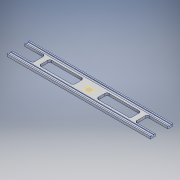
# Autodesk Inventor part: top
Saved by Autodesk Inventor 2017 (Build 210142000, 142)
## iProperties
Created: 2016-09-24
Part Number: top
Material: Aluminum 6061
Document SubType Name: Modeling
Designer: Kevin G
Density: 2.7 g/cm^3
Appearance: Aluminum - Flat
Author: Kevin G
Autodesk Inventor part; units mm, degrees
note: some values were not read from the file. Chosen so that the rebuilt part matches the saved one: direction of "Emboss7".
ref_plane "YZ Plane" through (0, 0, 0) normal (1, 0, 0) x (0, 1, 0)
ref_plane "XZ Plane" through (0, 0, 0) normal (0, 1, 0) x (-1, 0, 0)
ref_plane "XY Plane" through (0, 0, 0) normal (0, 0, 1) x (1, 0, 0)
sketch "Sketch1" plane through (0, 0, 0) normal (0, 0, 1) x (1, 0, 0)
  line L0 (-56.2006, 27.4418) -> (-175.6588, 27.4418)
  line L1 (-56.2006, -15.6625) -> (-175.6588, -15.6625)
  line L2 (-48.2006, -7.6625) -> (-48.2006, 19.4418)
  line L3 (-183.6588, -7.6625) -> (-183.6588, 19.4418)
  line L4 (-286.5288, -19.4915) -> (-213.2441, -19.4915)
  line L5 (-286.5288, 31.2885) -> (-213.2441, 31.2885)
  line L6 (-205.2441, 23.2885) -> (-205.2441, -11.4915)
  line L7 (51.9852, 27.4415) -> (171.5472, 27.4415)
  line L8 (51.9852, -15.6445) -> (171.5472, -15.6445)
  line L9 (43.9852, 19.4415) -> (43.9852, -7.6445)
  line L10 (179.5472, 19.4415) -> (179.5472, -7.6445)
  arc A0 (-205.2441, 23.2885) -> (-213.2441, 31.2885) centre (-213.2441, 23.2885) ccw
  arc A1 (-175.6588, 27.4418) -> (-183.6588, 19.4418) centre (-175.6588, 19.4418) ccw
  arc A2 (-183.6588, -7.6625) -> (-175.6588, -15.6625) centre (-175.6588, -7.6625) ccw
  arc A3 (-56.2006, -15.6625) -> (-48.2006, -7.6625) centre (-56.2006, -7.6625) ccw
  arc A4 (-48.2006, 19.4418) -> (-56.2006, 27.4418) centre (-56.2006, 19.4418) ccw
  arc A5 (-213.2441, -19.4915) -> (-205.2441, -11.4915) centre (-213.2441, -11.4915) ccw
  arc A6 (51.9852, 27.4415) -> (43.9852, 19.4415) centre (51.9852, 19.4415) ccw
  arc A7 (43.9852, -7.6445) -> (51.9852, -15.6445) centre (51.9852, -7.6445) ccw
  arc A8 (171.5472, -15.6445) -> (179.5472, -7.6445) centre (171.5472, -7.6445) ccw
  arc A9 (179.5472, 19.4415) -> (171.5472, 27.4415) centre (171.5472, 19.4415) ccw
  line L11 (-286.5288, 50.3385) -> (282.4312, 50.3385)
  line L12 (-286.5288, -38.5415) -> (282.4312, -38.5415)
  line L13 (-286.5288, 31.2885) -> (-286.5288, 50.3385)
  line L14 (-286.5288, -19.4915) -> (-286.5288, -38.5415)
  line L15 (179.5472, 5.8985) -> (201.1322, 5.9085)
  line L16 (282.4312, 31.2885) -> (209.1322, 31.2885)
  line L17 (201.1322, 23.2885) -> (201.1322, -11.4915)
  line L18 (209.1322, -19.4915) -> (282.4312, -19.4915)
  arc A10 (201.1322, -11.4915) -> (209.1322, -19.4915) centre (209.1322, -11.4915) ccw
  arc A11 (209.1322, 31.2885) -> (201.1322, 23.2885) centre (209.1322, 23.2885) ccw
  line L19 (282.4312, 50.3385) -> (282.4312, 31.2885)
  line L20 (282.4312, -19.4915) -> (282.4312, -38.5415)
  point P0 (0, 0)
  point P1 (0, 0)
  point P2 (-209.4751, 31.2885)
  point P3 (-205.2441, 26.6389)
  point P4 (-209.4751, -19.4915)
  point P5 (-179.9924, 27.4418)
  point P6 (-183.6588, 23.2495)
  point P7 (-183.6588, -11.4325)
  point P8 (-179.4288, -15.6625)
  point P9 (-48.2006, 23.2495)
  point P10 (-52.4306, 27.4418)
  point P11 (-52.9924, -15.6625)
  point P12 (-48.2006, -11.4325)
  point P13 (-205.2441, -15.2625)
  point P14 (48.2152, 27.4415)
  point P15 (43.9852, 23.2115)
  point P16 (48.2152, -15.6445)
  point P17 (179.5472, 23.2115)
  point P18 (175.3172, 27.4415)
  point P19 (175.3172, -15.6445)
  point P20 (179.5472, -11.4145)
  point P21 (43.9852, -11.4145)
  dimension "d0" = 135.4582
  dimension "d1" = 43.1043
  dimension "d4" = 21.5853
  dimension "d5" = 92.1858
  dimension "d8" = 8
  dimension "d9" = 8
  dimension "d10" = 8
  dimension "d50" = 50.7799
  dimension "d62" = 88.8799
  dimension "d63" = 19.05
  dimension "d64" = 50.7799
  constraints: 42 end point, 24 point on circle, 24 tangent, 20 point on line, 12 centre point, 9 vertical, 8 equal radius, 8 horizontal, 1 collinear, 1 midpoint, 1 perpendicular
  measures "d0" distance between parallel lines of L2 L3
  measures "d1" distance between parallel lines of L1 L0
  measures "d4" distance between parallel lines of L3 L6
  measures "d5" distance between parallel lines of L9 L2
  measures "d8" radius of A0
  measures "d9" radius of A1
  measures "d10" radius of A6
  measures "d50" distance between parallel lines of L5 L4
  measures "d62" distance between parallel lines of L12 L11
  measures "d63" distance between parallel lines of L11 L5
  measures "d64" distance between parallel lines of L16 L18
ref_plane "Work Plane7" through (0, 0, 9.525) normal (0, 0, 1) x (1, 0, 0)
extrude "Extrusion6" add sketch "Sketch1" along normal blind 9.525
sketch "Sketch7" plane through (0, 0, 9.525) normal (0, 0, 1) x (1, 0, 0)
  line L0 (-286.5288, 50.3385) -> (-286.5288, 31.2885) projected
  line L1 (282.4312, 31.2885) -> (282.4312, 50.3385) projected
  line L2 (-286.5288, 45.576) -> (282.4312, 45.576)
  line L3 (282.4312, 45.576) -> (282.4312, 36.051)
  line L4 (282.4312, 36.051) -> (-286.5288, 36.051)
  line L5 (-286.5288, 36.051) -> (-286.5288, 45.576)
  line L6 (282.4312, 50.3385) -> (-286.5288, 50.3385) projected
  line L7 (282.4312, -38.5415) -> (282.4312, -19.4915) projected
  line L8 (-286.5288, -24.254) -> (282.4312, -24.254)
  line L9 (282.4312, -24.254) -> (282.4312, -33.779)
  line L10 (282.4312, -33.779) -> (-286.5288, -33.779)
  line L11 (-286.5288, -33.779) -> (-286.5288, -24.254)
  line L12 (-286.5288, -38.5415) -> (282.4312, -38.5415) projected
  point P0 (0, 0)
  dimension "d98" = 9.525
  dimension "d99" = 4.7625
  dimension "d100" = 4.7625
  dimension "d101" = 9.525
  constraints: 16 end point, 4 parallel, 3 point on line, 2 horizontal, 2 perpendicular
  measures "d98" distance between parallel lines of L4 L2
  measures "d99" distance between parallel lines of L2 L6
  measures "d100" distance between parallel lines of L12 L10
  measures "d101" distance between parallel lines of L8 L10
emboss "Emboss7" sketch "Sketch7" operation cut depth 3 direction (0, 0, -1) contours L2 L1 L4 L0 | L10 L11 L8 L7
body "Solid5"
